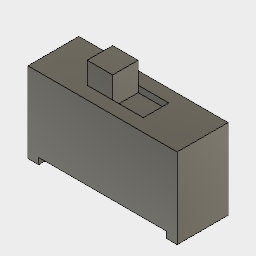
805 slide switch (Autodesk Fusion 360 design; units mm, degrees)
Autodesk Fusion 360 part; units mm, degrees
sketch "Sketch1" plane through (0, 0, 0) normal (0, 0, 1) x (1, 0, 0)
  line L0 (0, 0) -> (11.7, 0)
  line L1 (11.7, 0) -> (11.7, -4)
  line L2 (11.7, -4) -> (0, -4)
  line L3 (0, -4) -> (0, 0)
  line L4 (5.85, 0) -> (5.85, -4) construction
  line L5 (0, -2) -> (11.7, -2) construction
  line L6 (8.05, -3) -> (3.65, -3)
  line L7 (3.65, -3) -> (3.65, -1)
  line L8 (3.65, -1) -> (8.05, -1)
  line L9 (8.05, -1) -> (8.05, -3)
  line L10 (8.05, -3) -> (3.65, -1) construction
  line L11 (3.65, -3) -> (8.05, -1) construction
  line L12 (3.65, -1) -> (5.65, -1)
  line L13 (5.65, -1) -> (5.65, -3)
  line L14 (5.65, -3) -> (3.65, -3)
  line L15 (3.65, -3) -> (3.65, -1)
  point P0 (5.85, -2)
  dimension "d1" = 11.7
  dimension "d2" = 4
  dimension "d3" = 4.4
  dimension "d4" = 2
  dimension "d5" = 2
  measures "d1" distance of L0.start L0.end
  measures "d2" distance of L0.start L2.end
  measures "d3" distance of L7.end L8.end
  measures "d4" distance of L6.end L7.end
  measures "d5" distance of L7.end L12.end
extrude "Extrude1" add sketch "Sketch1" against normal blind 6.3 contours L0 L1 L2 L3 | L6 L8 L9 L13 | L6 L7 L8 L12 L13 L14 L15
extrude "Extrude2" cut sketch "Sketch1" against normal blind 0.5 contours L6 L8 L9 L13 | L6 L7 L8 L12 L13 L14 L15
extrude "Extrude3" add sketch "Sketch1" along normal blind 1.7 and the other way blind 0.5 contours L6 L7 L8 L12 L13 L14 L15
sketch "Sketch2" plane through (0, 0, -6.3) normal (0, 0, -1) x (1, 0, 0)
  line L0 (11.7, 4) -> (0, 4)
  line L1 (0, 4) -> (0, 0)
  line L2 (0, 0) -> (11.7, 0)
  line L3 (11.7, 0) -> (11.7, 4)
  line L4 (5.85, 4) -> (5.85, 0) construction
  line L5 (0, 2) -> (11.7, 2) construction
  line L6 (10.85, 0) -> (0.85, 0)
  line L7 (0.85, 0) -> (0.85, 4)
  line L8 (0.85, 4) -> (10.85, 4)
  line L9 (10.85, 4) -> (10.85, 0)
  line L10 (10.85, 0) -> (0.85, 4) construction
  line L11 (0.85, 0) -> (10.85, 4) construction
  point P0 (5.85, 2)
  dimension "d13" = 10
  dimension "d14" = 4
  measures "d13" distance of L7.end L8.end
  measures "d14" distance of L6.end L7.end
extrude "Extrude4" cut sketch "Sketch2" against normal blind 0.5 contours L0 L2 L6 L7 L8 L9
